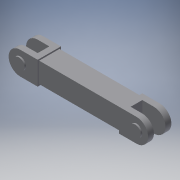
# Autodesk Inventor part: ShortArm
Saved by Autodesk Inventor 2018 (Build 220105000, 105)
## iProperties
Created: 2004-11-28
Document SubType Name: Modeling
Designer: Autodesk, Inc.
Manufacturer: Standard
Standards Organization: Custom
Description: SWING ARM, SHORT ARM
Mass: 540.311 g
Surface Area: 666.42 cm^2
Volume: 540.311 cm^3
Density: 1 g/cm^3
Material: Generic
Appearance: Default
CAGE: 1LJX3
Dept. ID: Product Design
Description #2: ---
Finish #1: ---
Finish #2: ---
Material ID: ---
Project Number: ---
Author: Autodesk, Inc.
Autodesk Inventor part; units mm, degrees
sketch "Sketch1" plane through (0, 0, 0) normal (0, 0, 1) x (1, 0, 0)
  line L0 (0, 25.4) -> (254, 25.4)
  line L1 (254, 25.4) -> (254, -25.4)
  line L2 (254, -25.4) -> (0, -25.4)
  line L3 (0, -25.4) -> (0, 25.4)
  circle A0 centre (0, 0) radius 25.4
  circle A1 centre (254, 0) radius 25.4
  dimension "d0" = 254
  dimension "d1" = 50.8
  constraints: 8 end point, 2 midpoint, 2 parallel, 2 vertical alignment, 1 coincident, 1 horizontal, 1 perpendicular, 4 other
  measures "d0" distance of L0.start L0.end
  measures "d1" distance of L0.end L1.end
extrude "Extrusion1" add sketch "Sketch1" along normal mid plane 50.8
sketch "Sketch2" plane through (0, 25.4, 25.4) normal (0, 1, 0) x (1, 0, 0)
  line L0 (-25.4, 50.8) -> (-25.4, 0) projected
  line L1 (-25.4, 50.8) -> (0, 50.8) projected
  line L2 (0, 0) -> (-25.4, 0) projected
  line L3 (0, 0) -> (254, 0) projected
  line L4 (254, 50.8) -> (0, 50.8) projected
  line L5 (-25.4, 12.7) -> (25.4, 12.7)
  line L6 (25.4, 12.7) -> (25.4, 38.1)
  line L7 (25.4, 38.1) -> (-25.4, 38.1)
  line L8 (-25.4, 38.1) -> (-25.4, 12.7)
  point P0 (-25.4, 25.4)
  point P1 (-25.4, 25.4)
  dimension "d4" = 25.4
  dimension "d10" = 50.8
  constraints: 8 end point, 2 midpoint, 2 parallel, 1 coincident, 1 horizontal, 1 perpendicular, 1 point on line
  measures "d4" distance of L5.end L6.end
  measures "d10" distance of L6.end L7.end
extrude "Extrusion2" cut sketch "Sketch2" against normal through all
ref_plane "Work Plane1" through (279.4, 0, 0) normal (1, 0, 0) x (0, 1, 0)
ref_plane "Work Plane2" through (-25.4, 0, 0) normal (1, 0, 0) x (0, 1, 0)
ref_plane "Work Plane3" through (127, 0, 0) normal (1, 0, 0) x (0, 1, 0)
sketch "Sketch5" plane through (0, 0, 25.4) normal (0, 0, 1) x (1, 0, 0)
  arc A0 (254, -25.4) -> (254, 25.4) centre (254, 0) ccw projected
  line L0 (0, 25.4) -> (254, 25.4) projected
  arc A1 (0, 25.4) -> (0, -25.4) centre (0, 0) ccw projected
  line L1 (254, -25.4) -> (0, -25.4) projected
  circle A2 centre (0, 0) radius 25.4 construction
  circle A3 centre (254, 0) radius 25.4 construction
  line L2 (38.1, 25.4) -> (38.1, -25.4)
  line L3 (215.9, 25.4) -> (215.9, -25.4)
  dimension "d11" = 12.7
  dimension "d13" = 12.7
  constraints: 4 end point, 4 point on line, 2 centre point, 2 coincident, 2 concentric, 2 perpendicular
  measures "d11" distance edge to line of A2 L2
  measures "d13" distance edge to line of A3 L3
extrude "Extrusion4" cut sketch "Sketch5" against normal blind 3.175 contours L1 L2 L0 L3
pattern_circular "Circular Pattern1" count 4 over 360 about axis through (-10, 0, 0) along (1, 0, 0) of "Extrusion4"
mirror "Mirror1" about plane through (127, 0, 0) normal (1, 0, 0) of "Extrusion2"
sketch "Sketch3" plane through (0, 0, 25.4) normal (0, 0, 1) x (1, 0, 0)
  arc A0 (0, 25.4) -> (0, -25.4) centre (0, 0) ccw projected
  arc A1 (254, -25.4) -> (254, 25.4) centre (254, 0) ccw projected
  circle A2 centre (0, 0) radius 12.7
  circle A3 centre (254, 0) radius 12.7
  dimension "d7" = 25.4
  constraints: 2 centre point, 2 coincident, 1 equal radius
  measures "d7" diameter of A2
extrude "Extrusion3" add sketch "Sketch3" along normal blind 3.175
mirror "Mirror2" about plane through (0, 0, 0) normal (0, 0, 1) of "Extrusion3"
equation "\"d13\" = d11"
body "Solid1"
